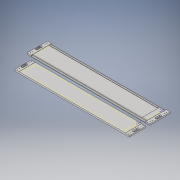
# Autodesk Inventor part: Fixture Base
Saved by Autodesk Inventor 2018 (Build 220112000, 112)
## iProperties
Created: 2016-04-07
Part Number: Fixture Base
Material: Generic
Document SubType Name: Modeling
Designer: Sam Clay
Density: 1 g/cm^3
Appearance: Default
Author: Sam Clay
Autodesk Inventor part; units mm, degrees
ref_plane "YZ Plane" through (0, 0, 0) normal (1, 0, 0) x (0, 1, 0)
ref_plane "XZ Plane" through (0, 0, 0) normal (0, 1, 0) x (-1, 0, 0)
ref_plane "XY Plane" through (0, 0, 0) normal (0, 0, 1) x (1, 0, 0)
sketch "Base Sketch" plane through (0, 0, 0) normal (0, 1, 0) x (-1, 0, 0)
  line L0 (0, 0) -> (1422.4, 0)
  line L1 (1422.4, 0) -> (1422.4, 254)
  line L2 (1320.8, 508) -> (0, 508)
  line L3 (0, 508) -> (0, 304.8)
  line L4 (0, 508) -> (-50.8, 508)
  line L5 (-50.8, 508) -> (-50.8, 304.8)
  line L6 (-50.8, 0) -> (0, 0)
  line L7 (0, 0) -> (0, 254)
  line L8 (1320.8, 508) -> (1371.6, 508)
  line L9 (1371.6, 508) -> (1371.6, 304.8)
  line L10 (1473.2, 0) -> (1422.4, 0)
  line L11 (1422.4, 0) -> (1422.4, 254)
  line L12 (1473.2, 254) -> (1473.2, 0)
  line L13 (-50.8, 254) -> (-50.8, 0)
  line L14 (1371.6, 304.8) -> (1320.8, 304.8)
  line L15 (1320.8, 304.8) -> (1320.8, 508)
  line L16 (1422.4, 254) -> (0, 254)
  line L17 (1320.8, 304.8) -> (0, 304.8)
  line L18 (0, 304.8) -> (-50.8, 304.8)
  line L19 (0, 254) -> (-50.8, 254)
  line L20 (0, 304.8) -> (0, 508)
  line L21 (0, 254) -> (0, 0)
  line L22 (1320.8, 304.8) -> (1320.8, 508)
  line L23 (1409.7, 0) -> (1409.7, 254)
  line L24 (12.7, 0) -> (12.7, 254)
  line L25 (1308.1, 304.8) -> (1308.1, 508) construction
  line L26 (12.7, 304.8) -> (12.7, 508) construction
  line L27 (1289.05, 323.85) -> (31.75, 323.85) construction
  line L28 (31.75, 323.85) -> (31.75, 488.95) construction
  line L29 (31.75, 488.95) -> (1289.05, 488.95) construction
  line L30 (1289.05, 488.95) -> (1289.05, 323.85) construction
  line L31 (1473.2, 254) -> (1422.4, 254)
  point P0 (-50.8, 254)
  point P1 (0, 254)
  dimension "d87" = 50.8
  dimension "d88" = 50.8
  dimension "d167" = 203.2
  dimension "d172" = 12.7
  dimension "d173" = 12.7
  dimension "d213" = 12.7
  dimension "d214" = 12.7
  dimension "d215" = 19.05
  dimension "d216" = 19.05
  dimension "d217" = 19.05
  dimension "d218" = 19.05
  dimension "d232" = 1524
  dimension "d233" = 50.8
  dimension "d234" = 50.8
  dimension "d235" = 1422.4
  dimension "d236" = 254
  dimension "d237" = 50.8
  constraints: 64 end point, 17 parallel, 14 perpendicular, 13 coincident, 12 point on line, 5 horizontal, 1 collinear
  measures "d87" distance of L6.end L6.start
  measures "d88" distance of L10.start L10.end
  measures "d167" distance between parallel lines of L2 L14
  measures "d172" distance between parallel lines of L23 L1
  measures "d173" distance between parallel lines of L21 L24
  measures "d213" distance between parallel lines of L22 L25
  measures "d214" distance between parallel lines of L3 L26
  measures "d215" distance between parallel lines of L27 L17
  measures "d216" distance between parallel lines of L25 L30
  measures "d217" distance between parallel lines of L26 L28
  measures "d218" distance between parallel lines of L2 L29
  measures "d232" distance between parallel lines of L12 L13
  measures "d233" distance between parallel lines of L9 L15
  measures "d234" distance between parallel lines of L5 L20
  measures "d235" distance between parallel lines of L9 L5
  measures "d236" distance between parallel lines of L16 L0
  measures "d237" distance between parallel lines of L14 L16
extrude "Lower Level" add sketch "Base Sketch" along normal blind 17.78 contours L6 L13 L19 L7 | L1 L31 L12 L10 | L8 L9 L14 L15 | L3 L18 L5 L4
extrude "Base" add sketch "Base Sketch" along normal blind 19.05 contours L7 L16 L24 L0 | L24 L16 L23 L0 | L23 L16 L1 L0 | L15 L17 L3 L2
sketch "Tracks Sketch" plane through (0, 19.05, 0) normal (0, 1, 0) x (1, 0, 0)
  line L0 (0, -254) -> (0, 0) projected
  line L1 (-1422.4, -19.812) -> (0, -19.812)
  line L2 (-1422.4, 0) -> (0, 0)
  line L3 (-1422.4, -234.188) -> (0, -234.188)
  line L4 (-1422.4, -254) -> (0, -254)
  line L5 (-63.5, -35.052) -> (-1422.4, -35.052)
  line L6 (-1422.4, -35.052) -> (-1422.4, -234.188)
  line L7 (-63.5, -234.188) -> (-63.5, -35.052)
  circle A0 centre (-67.31, -38.862) radius 8.89
  line L8 (-1371.6, -508) -> (50.8, -508) projected
  line L9 (50.8, -304.8) -> (-1371.6, -304.8) projected
  line L10 (-1473.2, -254) -> (50.8, -254) projected
  line L11 (50.8, 0) -> (-1473.2, 0) projected
  line L12 (-1371.6, -304.8) -> (-1371.6, -508) projected
  line L13 (50.8, -508) -> (50.8, -304.8) projected
  line L14 (-1473.2, 0) -> (-1473.2, -254) projected
  line L15 (50.8, -254) -> (50.8, 0) projected
  line L16 (-1422.4, 0) -> (-1422.4, -254) projected
  point P0 (-660.4, -254)
  point P1 (-1320.8, -254)
  dimension "d170" = 19.812
  dimension "d171" = 19.812
  dimension "d174" = 63.5
  dimension "d175" = 15.24
  dimension "d178" = 17.78
  dimension "d179" = 5.08
  dimension "d180" = 5.08
  dimension "d219" = 0
  dimension "d220" = 0
  constraints: 14 end point, 9 point on line, 5 perpendicular, 1 centre point, 1 horizontal, 1 parallel
  measures "d170" distance between parallel lines of L4 L3
  measures "d171" distance between parallel lines of L1 L2
  measures "d174" distance between parallel lines of L0 L7
  measures "d175" distance between parallel lines of L1 L5
  measures "d178" diameter of A0
  measures "d179" distance edge to line of A0 L5
  measures "d180" distance edge to line of A0 L7
  measures "d219" distance between parallel lines of L11 L2
  measures "d220" distance between parallel lines of L10 L4
extrude "Pocket side" cut sketch "Tracks Sketch" against normal blind 3.175 contours L3 L6 L5 A0 L7 | A0 L5 L7 | L7 L5 A0
extrude "Tracks" cut sketch "Tracks Sketch" against normal blind 12.7 contours L4 L16 L3 L0 | L1 L16 L2 L0
sketch "Handle Sketch" plane through (0, 17.78, 0) normal (0, 1, 0) x (1, 0, 0)
  line L0 (-1422.4, -35.052) -> (-1422.4, -19.812) projected
  line L1 (-1422.4, 0) -> (-1473.2, 0) projected
  line L2 (-1473.2, 0) -> (-1473.2, -254) projected
  line L3 (50.8, 0) -> (0, 0) projected
  line L4 (0, -19.812) -> (0, -234.188) projected
  line L5 (0, 0) -> (0, -19.812) projected
  line L6 (0, -234.188) -> (0, -254) projected
  line L7 (0, -254) -> (50.8, -254) projected
  line L8 (50.8, -254) -> (50.8, 0) projected
  line L9 (0, -508) -> (50.8, -508) projected
  line L10 (50.8, -508) -> (50.8, -304.8) projected
  line L11 (50.8, -304.8) -> (0, -304.8) projected
  line L12 (0, -304.8) -> (0, -508) projected
  line L13 (-1320.8, -508) -> (-1320.8, -304.8) projected
  line L14 (-1320.8, -304.8) -> (-1371.6, -304.8) projected
  line L15 (-1371.6, -304.8) -> (-1371.6, -508) projected
  line L16 (-1371.6, -508) -> (-1320.8, -508) projected
  line L17 (-1422.4, 0) -> (-1473.2, 0) construction
  line L18 (31.75, 0) -> (31.75, -508) construction
  line L19 (-1454.15, -88.9) -> (-1454.15, -165.1) construction
  line L20 (-1466.85, -101.6) -> (-1466.85, -152.4)
  line L21 (-1441.45, -152.4) -> (-1441.45, -101.6)
  arc A0 (-1441.45, -101.6) -> (-1466.85, -101.6) centre (-1454.15, -101.6) ccw
  arc A1 (-1466.85, -152.4) -> (-1441.45, -152.4) centre (-1454.15, -152.4) ccw
  line L22 (31.75, -88.9) -> (31.75, -165.1) construction
  line L23 (19.05, -101.6) -> (19.05, -152.4)
  line L24 (44.45, -152.4) -> (44.45, -101.6)
  arc A2 (44.45, -101.6) -> (19.05, -101.6) centre (31.75, -101.6) ccw
  arc A3 (19.05, -152.4) -> (44.45, -152.4) centre (31.75, -152.4) ccw
  line L25 (-1352.55, -368.3) -> (-1352.55, -444.5) construction
  line L26 (-1365.25, -381) -> (-1365.25, -431.8)
  line L27 (-1339.85, -431.8) -> (-1339.85, -381)
  arc A4 (-1339.85, -381) -> (-1365.25, -381) centre (-1352.55, -381) ccw
  arc A5 (-1365.25, -431.8) -> (-1339.85, -431.8) centre (-1352.55, -431.8) ccw
  line L28 (31.75, -368.3) -> (31.75, -444.5) construction
  line L29 (19.05, -381) -> (19.05, -431.8)
  line L30 (44.45, -431.8) -> (44.45, -381)
  arc A6 (44.45, -381) -> (19.05, -381) centre (31.75, -381) ccw
  arc A7 (19.05, -431.8) -> (44.45, -431.8) centre (31.75, -431.8) ccw
  line L31 (-1473.2, -254) -> (-1422.4, -254) projected
  line L32 (-1454.15, 0) -> (-1454.15, -254) construction
  line L33 (-1473.2, -254) -> (-1422.4, -254) construction
  line L34 (-1320.8, -304.8) -> (-1371.6, -304.8) construction
  line L35 (-1352.55, -304.8) -> (-1352.55, -508) construction
  line L36 (-1371.6, -508) -> (-1320.8, -508) construction
  line L37 (-1422.4, -254) -> (-1422.4, -35.052) projected
  line L38 (-1422.4, -19.812) -> (-1422.4, 0) projected
  point P0 (-1454.15, -25.4)
  point P1 (-1454.15, -50.8)
  point P2 (-1454.15, -203.2)
  point P3 (-1454.15, -228.6)
  point P4 (-1352.55, -317.5)
  point P5 (-1352.55, -342.9)
  point P6 (-1352.55, -469.9)
  point P7 (-1352.55, -495.3)
  point P8 (31.75, -495.3)
  point P9 (31.75, -469.9)
  point P10 (31.75, -342.9)
  point P11 (31.75, -317.5)
  point P12 (31.75, -228.6)
  point P13 (31.75, -203.2)
  point P14 (31.75, -50.8)
  point P15 (31.75, -25.4)
  point P16 (-1454.15, -127)
  point P17 (31.75, -127)
  point P18 (-1352.55, -406.4)
  point P19 (31.75, -406.4)
  dimension "d182" = 19.05
  dimension "d183" = 25.4
  dimension "d184" = 25.4
  dimension "d186" = 25.4
  dimension "d187" = 25.4
  dimension "d188" = 25.4
  dimension "d189" = 25.4
  dimension "d190" = 25.4
  dimension "d191" = 12.7
  dimension "d192" = 25.4
  dimension "d193" = 12.7
  dimension "d194" = 25.4
  dimension "d195" = 12.7
  dimension "d196" = 25.4
  dimension "d197" = 12.7
  dimension "d198" = 25.4
  dimension "d199" = 76.2
  dimension "d200" = 25.4
  dimension "d201" = 127
  dimension "d202" = 76.2
  dimension "d203" = 25.4
  dimension "d204" = 127
  dimension "d205" = 76.2
  dimension "d206" = 25.4
  dimension "d207" = 76.2
  dimension "d208" = 25.4
  dimension "d209" = 101.6
  dimension "d210" = 101.6
  dimension "d238" = 19.05
  dimension "d239" = 25.4
  dimension "d240" = 19.05
  constraints: 36 end point, 25 point on line, 24 point on circle, 16 tangent, 8 centre point, 5 midpoint, 4 parallel, 2 perpendicular, 1 horizontal, 15 other
  measures "d183" distance from line of point (-1454.15, -25.4) L1
  measures "d184" distance of point (-1454.15, -25.4) point (-1454.15, -50.8)
  measures "d186" distance of point (-1454.15, -203.2) point (-1454.15, -228.6)
  measures "d187" distance from line of point (31.75, -25.4) L3
  measures "d188" distance of point (31.75, -50.8) point (31.75, -25.4)
  measures "d189" distance from line of L7 point (31.75, -228.6)
  measures "d190" distance of point (31.75, -203.2) point (31.75, -228.6)
  measures "d191" distance from line of point (-1352.55, -317.5) L14
  measures "d192" distance of point (-1352.55, -342.9) point (-1352.55, -317.5)
  measures "d193" distance from line of L16 point (-1352.55, -495.3)
  measures "d194" distance of point (-1352.55, -469.9) point (-1352.55, -495.3)
  measures "d195" distance from line of L9 point (31.75, -495.3)
  measures "d196" distance of point (31.75, -469.9) point (31.75, -495.3)
  measures "d197" distance from line of point (31.75, -317.5) L11
  measures "d198" distance of point (31.75, -342.9) point (31.75, -317.5)
  measures "d199" distance of L19.start L19.end
  measures "d200" diameter of A1
  measures "d201" distance from line of L1 point (-1454.15, -127)
  measures "d202" distance of L22.start L22.end
  measures "d203" diameter of A3
  measures "d204" distance from line of L3 point (31.75, -127)
  measures "d205" distance of L25.start L25.end
  measures "d206" diameter of A5
  measures "d207" distance of L28.start L28.end
  measures "d208" diameter of A7
  measures "d209" distance from line of point (-1352.55, -406.4) L14
  measures "d210" distance from line of point (31.75, -406.4) L11
  measures "d238" distance between parallel lines of L32 L2
  measures "d239" distance of L32.end point (-1454.15, -228.6)
  measures "d240" distance between parallel lines of L35 L15
sketch "Origin Sketch" plane through (0, 19.05, 0) normal (0, 1, 0) x (1, 0, 0)
  line L0 (-1422.4, -35.052) -> (-75.3422, -35.052) construction
  line L1 (-12.7, 0) -> (-12.7, -254) construction
  line L2 (0, -304.8) -> (-1320.8, -304.8) construction
  line L3 (0, -304.8) -> (0, -508) construction
  line L4 (-12.7, -304.8) -> (-12.7, -508) construction
  line L5 (-1289.05, -323.85) -> (-31.75, -323.85) construction
  line L6 (-31.75, -488.95) -> (-1289.05, -488.95) construction
  line L7 (-31.75, -323.85) -> (-31.75, -488.95) construction
  line L8 (-1289.05, -488.95) -> (-1289.05, -323.85) construction
  line L9 (-1308.1, -304.8) -> (-1308.1, -508) construction
  line L10 (-1409.7, 0) -> (-1409.7, -254) construction
  line L11 (-63.5, -46.8942) -> (-63.5, -234.188) construction
  point P0 (-12.7, -35.052)
  point P1 (-25.4, -317.5)
  dimension "d211" = 12.7
  dimension "d212" = 25.4
  constraints: 2 point on line
  measures "d211" distance from line of L2 point (-25.4, -317.5)
  measures "d212" distance from line of L3 point (-25.4, -317.5)
extrude "Handles" cut sketch "Handle Sketch" along normal through all both and the other way through all contours A0 L21 A1 L20 | A2 L24 A3 L23 | A4 L27 A5 L26 | A6 L30 A7 L29
hole "Hole1" at (-1454.15, 17.78, 25.4) at (-1454.15, 17.78, 50.8) at (-1454.15, 17.78, 203.2) at (-1454.15, 17.78, 228.6) at (-1352.55, 17.78, 317.5) at (-1352.55, 17.78, 342.9) at (-1352.55, 17.78, 469.9) at (-1352.55, 17.78, 495.3) at (31.75, 17.78, 495.3) at (31.75, 17.78, 469.9) at (31.75, 17.78, 342.9) at (31.75, 17.78, 317.5) at (31.75, 17.78, 228.6) at (31.75, 17.78, 203.2) at (31.75, 17.78, 50.8) at (31.75, 17.78, 25.4) direction (0, -1, 0) diameter 6.35 end through all
body "Solid1"
